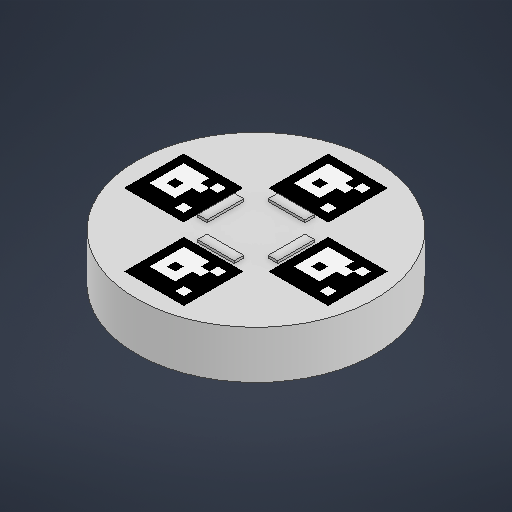
# Autodesk Inventor part: Spin Chuck
Saved by Autodesk Inventor 2025.1 (Build 291241000, 241)
## iProperties
Created: 2024-11-11
Part Number: Spin Chuck
Material: Generic
Document SubType Name: Modeling
Designer: jerem
Density: 1 g/cm^3
Appearance: Default
Author: jerem
Autodesk Inventor part; units mm, degrees
ref_plane "YZ Plane" through (0, 0, 0) normal (1, 0, 0) x (0, 1, 0)
ref_plane "XZ Plane" through (0, 0, 0) normal (0, 1, 0) x (-1, 0, 0)
ref_plane "XY Plane" through (0, 0, 0) normal (0, 0, 1) x (1, 0, 0)
sketch "Sketch1" plane through (0, 0, 0) normal (0, 1, 0) x (-1, 0, 0)
  line L0 (-12.7, 12.7) -> (12.7, 12.7)
  line L1 (12.7, 12.7) -> (12.7, -12.7)
  line L2 (12.7, -12.7) -> (-12.7, -12.7)
  line L3 (-12.7, -12.7) -> (-12.7, 12.7)
  line L4 (-12.7, 12.7) -> (12.7, -12.7) construction
  line L5 (12.7, 12.7) -> (-12.7, -12.7) construction
  circle A0 centre (0, 0) radius 50
  line L6 (12.8, -7.7) -> (16.8, -7.7)
  line L7 (16.8, -7.7) -> (16.8, 7.7)
  line L8 (16.8, 7.7) -> (12.8, 7.7)
  line L9 (12.8, 7.7) -> (12.8, -7.7)
  line L10 (-12.5, -17.7) -> (12.5, -17.7) construction
  line L11 (12.5, -17.7) -> (12.5, -42.7) construction
  line L12 (12.5, -42.7) -> (-12.5, -42.7) construction
  line L13 (-12.5, -42.7) -> (-12.5, -17.7) construction
  line L14 (0, -12.7) -> (0, -17.7) construction
  line L15 (17.8, 12.5) -> (42.8, 12.5) construction
  line L16 (42.8, 12.5) -> (42.8, -12.5) construction
  line L17 (42.8, -12.5) -> (17.8, -12.5) construction
  line L18 (17.8, -12.5) -> (17.8, 12.5) construction
  line L19 (-42.7, 12.5) -> (-17.7, 12.5) construction
  line L20 (-17.7, 12.5) -> (-17.7, -12.5) construction
  line L21 (-17.7, -12.5) -> (-42.7, -12.5) construction
  line L22 (-42.7, -12.5) -> (-42.7, 12.5) construction
  line L23 (-12.5, 42.7) -> (12.5, 42.7) construction
  line L24 (12.5, 42.7) -> (12.5, 17.7) construction
  line L25 (12.5, 17.7) -> (-12.5, 17.7) construction
  line L26 (-12.5, 17.7) -> (-12.5, 42.7) construction
  line L27 (17.8, 0) -> (12.8, 0) construction
  line L28 (-12.7, 0) -> (-17.7, 0) construction
  line L29 (0, 17.7) -> (0, 12.7) construction
  point P0 (30.3, 12.5)
  point P1 (-30.2, 12.5)
  point P2 (0, 42.7)
  dimension "d0" = 25.4
  dimension "d1" = 25.4
  dimension "d2" = 0.1
  dimension "d3" = 4
  dimension "d4" = 100
  dimension "d7" = 5
  dimension "d8" = 5
  dimension "d21" = 25
  dimension "d28" = 25
  dimension "d35" = 25
  dimension "d44" = 25
  dimension "d73" = 5
  dimension "d74" = 5
  dimension "d75" = 5
  dimension "d76" = 5
  constraints: 28 end point, 13 midpoint, 5 perpendicular, 4 horizontal, 4 parallel, 2 vertical, 1 centre point, 1 coincident, 8 other
  measures "d0" distance of L1.end L2.end
  measures "d1" distance of L0.end L1.end
  measures "d2" distance between parallel lines of L1 L9
  measures "d3" distance of L7.end L8.end
  measures "d4" diameter of A0
  measures "d7" distance between parallel lines of L2 L6
  measures "d8" distance between parallel lines of L0 L8
  measures "d21" distance of L10.start L10.end
  measures "d28" distance of L18.end L16.start
  measures "d35" distance of L22.end L20.start
  measures "d44" distance of L26.end L24.start
  measures "d73" distance between parallel lines of L25 L0
  measures "d74" distance of L14.start L14.end
  measures "d75" distance of L28.start L28.end
  measures "d76" distance of L27.start L27.end
extrude "Extrusion1" add sketch "Sketch1" against normal blind 20 contours L0 L1 L2 L3 | A0 | L9 L8 L7 L6
extrude "Extrusion2" add sketch "Sketch1" along normal blind 1 contours L9 L8 L7 L6
pattern_circular "Circular Pattern1" count 4 over 360 about axis through (0, 0, 0) along (0, -1, 0) of "Extrusion2"
decal "Decal1"
decal "Decal2"
decal "Decal3"
decal "Decal4"
equation "\"d8\" = d7"
equation "\"d73\" = d74"
equation "\"d75\" = d74"
equation "\"d76\" = d74"
body "Solid1"
